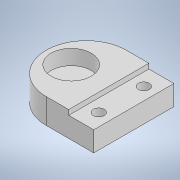
# Autodesk Inventor part: Деталь основы рулевого управления
Saved by Autodesk Inventor 2020 (Build 240168000, 168)
## iProperties
Created: 2021-06-17
Part Number: Деталь основы рулевого управления
Material: Типовые
Document SubType Name: Modeling
Designer: Антон
Density: 1 g/cm^3
Appearance: По умолчанию
Author: Антон
Autodesk Inventor part; units mm, degrees
ref_plane "YZ Plane" through (0, 0, 0) normal (1, 0, 0) x (0, 1, 0)
ref_plane "XZ Plane" through (0, 0, 0) normal (0, 1, 0) x (-1, 0, 0)
ref_plane "XY Plane" through (0, 0, 0) normal (0, 0, 1) x (1, 0, 0)
sketch "Эскиз1" plane through (0, 0, 0) normal (0, 1, 0) x (-1, 0, 0)
  line L0 (0, 0) -> (17.5, 0)
  line L1 (17.5, 0) -> (17.5, -16)
  line L2 (17.5, -16) -> (0, -16)
  line L3 (0, -16) -> (0, 0)
  dimension "d0" = 17.5
  dimension "d1" = 16
  constraints: 8 end point, 2 parallel, 1 horizontal, 1 perpendicular
  measures "d0" distance of L1.end L2.end
  measures "d1" distance of L0.end L1.end
extrude "Выдавливание1" add sketch "Эскиз1" along normal blind 5
sketch "Эскиз2" plane through (0, 5, 0) normal (0, 1, 0) x (1, 0, 0)
  line L0 (-17.5, 16) -> (-17.5, 0) projected
  line L1 (-17.5, 8) -> (-12.5, 8)
  circle A0 centre (-12.5, 8) radius 4
  point P0 (0, 0)
  dimension "d4" = 5
  dimension "d5" = 8
  constraints: 2 end point, 1 centre point, 1 coincident, 1 horizontal, 1 midpoint
  measures "d4" distance of L1.start L1.end
  measures "d5" diameter of A0
extrude "Выдавливание2" cut sketch "Эскиз2" against normal blind 3
fillet "Сопряжение1" radius 8 2 edges at (-17.5, 2.5, 0) (-17.5, 2.5, -16)
sketch "Эскиз3" plane through (0, 0, 0) normal (0, -1, 0) x (1, 0, 0)
  line L0 (0, 0) -> (0, -16) projected
  line L1 (0, -8) -> (-2.5, -8)
  line L2 (-2.5, -3.5) -> (-2.5, -12.5)
  dimension "d9" = 2.5
  dimension "d10" = 9
  constraints: 4 end point, 2 midpoint, 1 horizontal, 1 perpendicular
  measures "d9" distance of L1.end L1.start
  measures "d10" distance of L2.start L2.end
hole "Отверстие1" at (-2.5, 0, -3.5) at (-2.5, 0, -12.5) direction (0, 1, 0) diameter 2.2 end through all countersink diameter 4.5 countersink angle 90
sketch "Эскиз4" plane through (0, 5, 0) normal (0, 1, 0) x (1, 0, 0)
  line L0 (0, 0) -> (-5, 0)
  line L1 (-5, 0) -> (-5, 16)
  line L2 (-5, 16) -> (0, 16)
  line L3 (0, 16) -> (0, 0)
  line L4 (0, 16) -> (-9.5, 16) projected
  dimension "d18" = 5
  constraints: 8 end point, 2 parallel, 1 collinear, 1 horizontal, 1 perpendicular
  measures "d18" distance between parallel lines of L3 L1
extrude "Выдавливание3" cut sketch "Эскиз4" against normal blind 1
